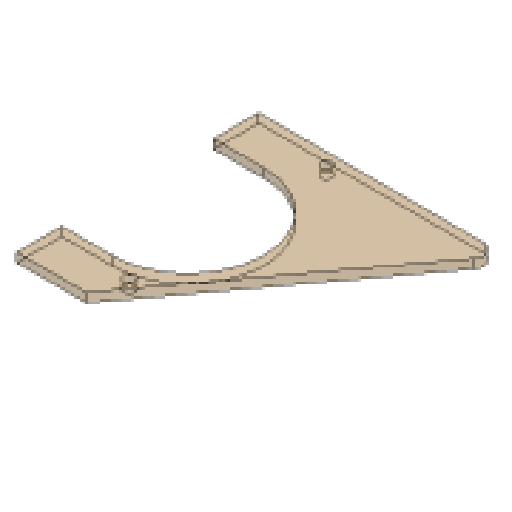
# Autodesk Inventor part: FoldedGuides
Saved by Autodesk Inventor 2023 (Build 270158000, 158)
## iProperties
Created: 2022-11-11
Part Number: FoldedGuides
Material: Polycarbonate, Smoke
Document SubType Name: Modeling
Designer: deli
Density: 1.2 g/cm^3
Appearance: Polycarbonate - Smoked
Author: deli
Autodesk Inventor part; units mm, degrees
ref_plane "YZ Plane" through (0, 0, 0) normal (1, 0, 0) x (0, 1, 0)
ref_plane "XZ Plane" through (0, 0, 0) normal (0, 1, 0) x (-1, 0, 0)
ref_plane "XY Plane" through (0, 0, 0) normal (0, 0, 1) x (1, 0, 0)
sketch "Sketch1" plane through (0, 0, 0) normal (0, 1, 0) x (-1, 0, 0)
  line L0 (-91.7866, -63.4215) -> (-91.7866, -79.4215)
  line L1 (-159.7033, -116.0004) -> (-112.7525, -63.4215)
  circle A0 centre (-183.9616, -81.2095) radius 41.267 construction
  line L2 (-112.7525, -63.4215) -> (-91.7866, -63.4215)
  line L3 (-112.7525, -63.4215) -> (-91.7866, -39.9425)
  line L4 (-91.7866, -39.9425) -> (-91.7866, -63.4215)
  line L5 (-109.6116, -133.3215) -> (-91.7866, -133.3215)
  line L6 (-91.7866, -133.3215) -> (-91.7866, -149.3215)
  line L7 (-91.7866, -149.3215) -> (-144.7854, -149.3215)
  line L8 (-109.6116, -79.4215) -> (-91.7866, -79.4215)
  arc A1 (-109.6116, -79.4215) -> (-109.6116, -133.3215) centre (-109.6116, -106.3715) ccw
  circle A2 centre (-119.7866, -145.3215) radius 1.939
  circle A3 centre (-119.7866, -75.3215) radius 2
  arc A4 (-159.7033, -116.0004) -> (-144.7854, -149.3215) centre (-144.7854, -129.3215) ccw
  point P0 (0, 0)
  point P1 (-91.7866, -54.2052)
  point P2 (-103.5347, -53.0989)
  dimension "d4" = 82.534
  dimension "d6" = 92.175
  dimension "d12" = 16
  dimension "d15" = 16
  dimension "d16" = 85.9
  dimension "d17" = 17.825
  dimension "d18" = 4
  dimension "d20" = 4
  dimension "d21" = 28
  dimension "d22" = 28
  dimension "d27" = 70
  dimension "d29" = 40
  dimension "d31" = 4
  dimension "d33" = 41.267
  constraints: 18 end point, 5 centre point, 5 tangent, 4 point on circle, 3 collinear, 3 perpendicular, 2 point on line, 1 horizontal, 1 vertical
  measures "d4" diameter of A0
  measures "d6" distance from line of L0 A0.centre
  measures "d12" distance between parallel lines of L5 L7
  measures "d15" distance between parallel lines of L2 L8
  measures "d16" distance between parallel lines of L2 L7
  measures "d17" distance from line of A1.centre L0
  measures "d18" diameter of A3
  measures "d20" distance from line of L7 A2.centre
  measures "d21" distance from line of L6 A2.centre
  measures "d22" distance from line of L0 A3.centre
  measures "d27" distance of A2.centre A3.centre
  measures "d29" diameter of A4
  measures "d31" distance edge to line of A1 L1
  measures "d33" vertical distance of L3.end A0.centre
extrude "Extrusion1" add sketch "Sketch1" along normal blind 3.175
equation "\"d15\" = d12"
equation "\"d22\" = d21"
equation "\"d33\" = 0.5 * d4"
body "Solid1"
